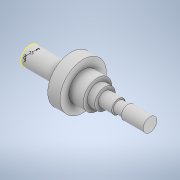
# Autodesk Inventor part: Part1
Saved by Autodesk Inventor 2021 (Build 250183000, 183)
## iProperties
Created: 2020-12-31
Part Number: Part1
Material: Generic
Document SubType Name: Modeling
Designer: dieku
Density: 1 g/cm^3
Appearance: Default
Author: dieku
Autodesk Inventor part; units mm, degrees
ref_plane "YZ Plane" through (0, 0, 0) normal (1, 0, 0) x (0, 1, 0)
ref_plane "XZ Plane" through (0, 0, 0) normal (0, 1, 0) x (-1, 0, 0)
ref_plane "XY Plane" through (0, 0, 0) normal (0, 0, 1) x (1, 0, 0)
sketch "Sketch1" plane through (0, 0, 0) normal (0, 0, 1) x (1, 0, 0)
  line L0 (0, 0) -> (0, 13.5)
  line L1 (0, 13.5) -> (60, 13.5)
  line L2 (60, 13.5) -> (60, 0) construction
  line L3 (60, 0) -> (60, 34)
  line L4 (60, 34) -> (78, 34)
  line L5 (78, 34) -> (78, 0)
  line L6 (78, 0) -> (78, 21)
  line L7 (78, 21) -> (99, 21)
  line L8 (99, 21) -> (99, 0)
  line L9 (99, 0) -> (99, 15)
  line L10 (99, 15) -> (110, 15)
  line L11 (110, 15) -> (110, 0)
  line L12 (110, 0) -> (110, 10)
  line L13 (110, 10) -> (130, 10)
  line L14 (130, 10) -> (130, 0)
  line L15 (130, 0) -> (130, 8)
  line L16 (130, 8) -> (144, 8)
  line L17 (144, 8) -> (144, 0)
  line L18 (144, 0) -> (144, 10)
  line L19 (144, 10) -> (176, 10)
  line L20 (176, 10) -> (176, 0)
  line L21 (0, 0) -> (291.3618, 0) construction
  line L22 (0, 0) -> (176, 0)
  line L23 (47.9027, 0) -> (47.9027, 4) construction
  line L24 (60, 4) -> (56.5, 4) construction
  line L25 (52.5, 4) -> (40.5, 4)
  line L26 (36.5, 4) -> (33, 4) construction
  line L27 (33, 4) -> (0, 4) construction
  line L28 (46.5, 4) -> (46.5, 2) construction
  line L29 (46.5, 2) -> (40.5, 2) construction
  arc A0 (40.5, 4) -> (40.5, -4) centre (40.5, 0) ccw
  line L30 (46.5, 2) -> (52.5, 2) construction
  arc A1 (52.5, -4) -> (52.5, 4) centre (52.5, 0) ccw
  line L31 (40.5, -4) -> (52.5, -4)
  dimension "d4" = 13.5
  dimension "d5" = 60
  dimension "d9" = 18
  dimension "d10" = 21
  dimension "d11" = 21
  dimension "d12" = 15
  dimension "d13" = 11
  dimension "d14" = 10
  dimension "d15" = 20
  dimension "d16" = 8
  dimension "d17" = 14
  dimension "d18" = 10
  dimension "d19" = 32
  dimension "d28" = 3.5
  dimension "d29" = 20
  dimension "d30" = 3.5
  dimension "d31" = 6
  dimension "d32" = 8
  dimension "d33" = 6
  dimension "d34" = 8
  constraints: 64 end point, 14 perpendicular, 11 point on line, 6 horizontal, 5 vertical, 4 point on circle, 2 centre point, 1 midpoint, 1 parallel, 1 tangent
  measures "d4" distance of L0.start L0.end
  measures "d5" distance of L0.end L1.end
  measures "d9" distance of L3.end L4.end
  measures "d10" distance of L5.end L6.end
  measures "d11" distance of L6.end L7.end
  measures "d12" distance of L8.end L9.end
  measures "d13" distance of L9.end L10.end
  measures "d14" distance of L11.end L12.end
  measures "d15" distance of L12.end L13.end
  measures "d16" distance of L14.end L15.end
  measures "d17" distance of L15.end L16.end
  measures "d18" distance of L17.end L18.end
  measures "d19" distance of L18.end L19.end
  measures "d28" distance of L24.start L24.end
  measures "d29" distance of L24.end L26.start
  measures "d30" distance of L26.start L26.end
  measures "d31" distance of L28.end L29.end
  measures "d32" diameter of A0
  measures "d33" distance of L28.end L30.end
  measures "d34" diameter of A1
revolve "Revolution1" add sketch "Sketch1" angle 360 about axis through (0, 0, 0) along (1, 0, 0) contours L0 L1 L3 L22 A1 L25 A0 | A0 L25 A1 L22 | L3 L4 L5 L22 | L5 L7 L8 L22 | L8 L10 L11 L22 | L11 L13 L14 L22 | L14 L16 L17 L22 | L17 L18 L19 L20 L22
sketch "Sketch2" plane through (0, 0, 0) normal (-1, 0, 0) x (0, 0, 1)
  circle A0 centre (0, 0) radius 13.5 projected
  line L0 (-13.5, 0) -> (9.5, 0) construction
  line L1 (9.5, 0) -> (9.5, 4) construction
  line L2 (9.5, 0) -> (9.5, -4) construction
  dimension "d21" = 23
  dimension "d22" = 4
  dimension "d23" = 4
  constraints: 6 end point, 2 vertical, 1 horizontal, 1 horizontal alignment, 1 other
  measures "d21" distance of L0.start L0.end
  measures "d22" distance of L0.end L1.end
  measures "d23" distance of L0.end L2.end
body "Solid1"
